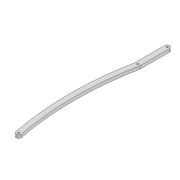
# Autodesk Inventor part: Part_7
Saved by Autodesk Inventor 2022 (Build 260153000, 153)
## iProperties
Created: 2022-04-22
Part Number: Part_7
Material: Generic
Document SubType Name: Modeling
Designer: dell
Density: 1 g/cm^3
Appearance: Default
Mass: 3.65128 g
Surface Area: 31.7858 cm^2
Volume: 3.65128 cm^3
Author: dell
Autodesk Inventor part; units mm, degrees
ref_plane "YZ Plane" through (0, 0, 0) normal (1, 0, 0) x (0, 1, 0)
ref_plane "XZ Plane" through (0, 0, 0) normal (0, 1, 0) x (-1, 0, 0)
ref_plane "XY Plane" through (0, 0, 0) normal (0, 0, 1) x (1, 0, 0)
sketch "Sketch1" plane through (0, 0, 0) normal (0, 1, 0) x (-1, 0, 0)
  line L0 (0, 0) -> (0, -288.984) construction
  line L1 (5, 0) -> (5, -288.984)
  line L2 (-5, -288.984) -> (-5, 0)
  arc A0 (5, 0) -> (-5, 0) centre (0, 0) ccw
  arc A1 (-5, -288.984) -> (5, -288.984) centre (0, -288.984) ccw
  circle A2 centre (0, 0) radius 1.65
  circle A3 centre (0, -288.984) radius 1.65
  circle A4 centre (0, -231.585) radius 1.65
  arc A5 (-5, -231.585) -> (-5, 0) centre (-593.7207, -115.7925) ccw
  arc A6 (5, -231.585) -> (5, 0) centre (-583.7207, -115.7925) ccw
  point P0 (0, -144.492)
  dimension "d0" = 3.3
  dimension "d1" = 3.3
  dimension "d2" = 10
  dimension "d3" = 288.984
  dimension "d14" = 3.3
  dimension "d15" = 231.585
  dimension "d18" = 600
  dimension "d19" = 600
  constraints: 8 end point, 8 point on circle, 7 centre point, 4 tangent, 3 point on line, 2 coincident, 2 horizontal alignment, 1 midpoint, 1 parallel, 1 vertical
  measures "d0" diameter of A2
  measures "d1" diameter of A3
  measures "d2" distance between parallel lines of L2 L1
  measures "d3" distance of L0.end L0.start
  measures "d14" diameter of A4
  measures "d15" distance of L0.start A4.centre
  measures "d18" radius of A5
  measures "d19" radius of A6
extrude "Extrusion1" add sketch "Sketch1" along normal blind 6 contours L1 A1 L2 A5 | L1 A5 A6 | L1 A5 A0
body "Solid1"
